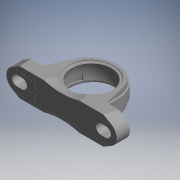
# Autodesk Inventor part: housingSYWK 506 Y-h
Saved by Autodesk Inventor 2017.3 (Build 213256000, 256)
## iProperties
Part Number: housingSYWK 506 Y-h
Material: Generic
Catalog Web Link: www.cadenas.de
Description: ayp_001_hc_hh_hy-ayl_001_hp_housing-Plummer block housings for Y-bearings
Vendor: SKF
Document SubType Name: Modeling
Designer: partserver
Manufacturer: SKF
Mass: 127.227 g
Surface Area: 312.414 cm^2
Volume: 127.227 cm^3
Density: 1 g/cm^3
Appearance: PSOLRGB-175-175-175
Category: PARTsolutions
Company: SKF
Title: housingSYWK 506 Y-h
Author: Cadenas PARTsolutions
Comments: Plummer block housings for Y-bearings
PSOL_IDENT_0: {$CADENAS_DATA\23d-libs\skf\bearings_units_and_housings\bearing_units\ball_bearing_units\y-units\y-b
PSOL_IDENT_1: earing_plummer_block_units_parts\ayp_001_hc_hh_hy-ayl_001_hp_housing.prj},217 {VTYP=3D},{NB=housingS
PSOL_IDENT_2: YWK 506 Y-h},{LINA=housingSYWK 506 Y-h},{NN=ayp_001_hc_hh_hy-ayl_001_hp_housing},{DATE=20.09.2021 12
PSOL_IDENT_3: :02:20},{GEOMDATE=16.12.2020 09:20:11},{VERSION=},{LINEID=5570},{WBVAR=ENDCOVER},{WBNUMERIC=}  {NB=h
PSOL_IDENT_4: ousingSYWK 506 Y-h},{LINA=housingSYWK 506 Y-h},{KT=DUMMY},{DESIGNATION=SYWK 506 Y},{DESIGN=sywk},{EN
PSOL_IDENT_5: DCOVER=},{ECPN=},{D=62.000},{H1=42.900},{A=40.000},{A1=25.000},{A5=30.500},{H=82.000},{H2=19.000},{J=
PSOL_IDENT_6: 121.000},{L=159.000},{N=21.500},{N1=14.500},{RG=},{R1=MIN},{RA=MIN},{DN=MIN},{SWN=MIN},{GN=},{J6=MIN
PSOL_IDENT_7: },{J7=MIN},{N4=MIN},{MASS=0.210},{G=12.000},{GIN=0.500},{COVER=ECW 206},{PIM=SYWK 506 Y},{LOOKUP=AEC
PSOL_IDENT_8: ALG,DECALG,D1ECALG,D2ECALG},{AEC=33.500},{AECALG=COVER,HEL02,AEC},{DEC=54.100},{DECALG=COVER,HED10,D
PSOL_IDENT_9: EC},{D1EC=64.400},{D1ECALG=COVER,HED13,D1EC},{D2EC=66.000},{D2ECALG=COVER,HED12,D2EC},{PPATH=apb_001
PSOL_IDENT_10: -002_apf_001_app_001_asmtpl.prj},{HIDE=0},{COPYTABLE=apb_001-002_apf_001_app_001_dummy|DUMMY,apb_001
PSOL_IDENT_11: -002_apf_001_app_001_housing|HOUSING,apb_001-002_apf_001_app_001_housing_arc|HOUSING2},{DUMMY=dummy}
PSOL_IDENT_12: ,{HOUSING=housing},{HOUSING2=housing2},{CANGLE=79.258},{ACRL=31.985},{ARCC=5.393},{S=0},{NON=},{DS=0
PSOL_IDENT_13: .000},{NOCUT=},{H3=MIN},{JMAX=128.000},{JMIN=114.000},{A5UP=31.000},{L1=MIN},{H4=MIN},{R2=MIN},{L2=M
PSOL_IDENT_14: IN},{H5=MIN},{L6=MIN},{L7=MIN},{H6=MIN},{L8=MIN},{R3=MIN},{L9=MIN},{ANG=MIN},{L10=MIN},{H7=MIN},{H8=
PSOL_IDENT_15: MIN},{R4=MIN},{R5=MIN},{R6=MIN},{H9=MIN},{ANG1=MIN},{ANG2=MIN},{L11=MIN},{R7=MIN},{L12=MIN},{R8=MIN}
PSOL_IDENT_16: ,{L13=MIN},{H10=MIN},{H11=MIN},{L14=MIN},{R9=MIN},{L15=MIN},{H12=MIN},{L16=MIN},{L17=MIN},{DRAFT=MIN
PSOL_IDENT_17: },{SCALE=MIN}
NB: housingSYWK 506 Y-h
NN: ayp_001_hc_hh_hy-ayl_001_hp_housing
NT: Plummer block housings for Y-bearings
NBSYN: $HOUSING.$DESIGNATION.$ECPN.-h
LINA: housingSYWK 506 Y-h
CATALOG: SKF
DESIGNATION: SYWK 506 Y
DESIGN: sywk
ENDCOVER: w/o End Cover
D: 62
H1: 42.9
A: 40
A1: 25
A5: 30.5
H: 82
H2: 19
J: 121
L: 159
N: 21.5
N1: 14.5
R1: 0
RA: 0
DN: 0
SWN: 0
J6: 0
J7: 0
N4: 0
MASS: 0.21
G: 12
GIN: 0.5
COVER: ECW 206
PIM: SYWK 506 Y
AEC: 33.5
DEC: 54.1
D1EC: 64.4
D2EC: 66
DS: 0
H3: 0
JMAX: 128
JMIN: 114
A5UP: 31
L1: 0
H4: 0
R2: 0
L2: 0
H5: 0
L6: 0
L7: 0
H6: 0
L8: 0
R3: 0
L9: 0
ANG: 0
L10: 0
H7: 0
H8: 0
R4: 0
R5: 0
R6: 0
H9: 0
ANG1: 0
ANG2: 0
L11: 0
R7: 0
L12: 0
R8: 0
L13: 0
H10: 0
H11: 0
L14: 0
R9: 0
L15: 0
H12: 0
L16: 0
L17: 0
DRAFT: 0
SCALE: 0
SUPPLIER: SKF
ARTICLENO: housingSYWK 506 Y-h
BOMINFO: housingSYWK 506 Y-h
CREATOR: CADENAS GmbH
Autodesk Inventor part; units mm, degrees
ref_plane "YZ Plane" through (0, 0, 0) normal (1, 0, 0) x (0, 1, 0)
ref_plane "XZ Plane" through (0, 0, 0) normal (0, 1, 0) x (-1, 0, 0)
ref_plane "XY Plane" through (0, 0, 0) normal (0, 0, 1) x (1, 0, 0)
sketch "Sketch_1" plane through (0, 0, 0) normal (1, 0, 0) x (0, 1, 0)
  line L0 (0, -20) -> (0, 20)
  line L1 (35.7991, 20) -> (32.5, 14.2857)
  line L2 (32.5, 14.2857) -> (32.5, 13.2857)
  arc A0 (31.5, 12.2857) -> (32.5, 13.2857) centre (31.5, 13.2857) ccw
  line L3 (31.5, 12.2857) -> (28.9616, 12.2857)
  line L4 (28.9616, 12.2857) -> (28.6105, 11.9347)
  arc A1 (28.6105, -11.9347) -> (28.6105, 11.9347) centre (0, 0) ccw
  line L5 (28.6105, -11.9347) -> (28.9616, -12.2857)
  line L6 (28.9616, -12.2857) -> (31.5, -12.2857)
  arc A2 (32.5, -13.2857) -> (31.5, -12.2857) centre (31.5, -13.2857) ccw
  line L7 (32.5, -13.2857) -> (32.5, -14.2857)
  line L8 (32.5, -14.2857) -> (35.7991, -20)
  line L9 (35.7991, -20) -> (119.25, -20)
  line L10 (119.25, -20) -> (119.25, 20)
  line L11 (119.25, 20) -> (35.7991, 20)
  constraints: 24 end point, 6 point on circle, 3 centre point
revolve "Revolution1" add sketch "Sketch_1" angle 360 about axis through (0, 0, -20) along (0, 0, -1)
sketch "Sketch_2" plane through (0, 0, 0) normal (0, 0, 1) x (1, 0, 0)
  circle A0 centre (0, 0) radius 119.25
  line L0 (-79.5, -23.9) -> (-79.5, -42.9)
  line L1 (-79.5, -42.9) -> (79.5, -42.9)
  line L2 (79.5, -42.9) -> (79.5, -23.9)
  line L3 (79.5, -23.9) -> (49.75, -23.9)
  arc A1 (44.9663, -20.3546) -> (49.75, -23.9) centre (49.75, -18.9) ccw
  line L4 (44.9663, -20.3546) -> (35.4954, 10.7929)
  arc A2 (35.4954, 10.7929) -> (-35.4954, 10.7929) centre (0, 0) ccw
  line L5 (-35.4954, 10.7929) -> (-44.9663, -20.3546)
  arc A3 (-49.75, -23.9) -> (-44.9663, -20.3546) centre (-49.75, -18.9) ccw
  line L6 (-49.75, -23.9) -> (-79.5, -23.9)
  constraints: 14 end point, 6 point on circle, 4 centre point
extrude "Extrusion1" cut sketch "Sketch_2" along normal mid plane 40
sketch "Sketch_3" plane through (0, 0, 0) normal (0, 1, 0) x (-1, 0, 0)
  line L0 (87.45, -22) -> (87.45, 22)
  line L1 (87.45, 22) -> (-87.45, 22)
  line L2 (-87.45, 22) -> (-87.45, -22)
  line L3 (-87.45, -22) -> (87.45, -22)
  arc A0 (71.75, -13.4234) -> (71.75, 13.4234) centre (64, 0) ccw
  line L4 (71.75, 13.4234) -> (61.5192, 19.3301)
  arc A1 (61.5192, 19.3301) -> (59.0192, 20) centre (59.0192, 15) ccw
  line L5 (59.0192, 20) -> (-59.0192, 20)
  arc A2 (-59.0192, 20) -> (-61.5192, 19.3301) centre (-59.0192, 15) ccw
  line L6 (-61.5192, 19.3301) -> (-71.75, 13.4234)
  arc A3 (-71.75, 13.4234) -> (-71.75, -13.4234) centre (-64, 0) ccw
  line L7 (-71.75, -13.4234) -> (-61.5192, -19.3301)
  arc A4 (-61.5192, -19.3301) -> (-59.0192, -20) centre (-59.0192, -15) ccw
  line L8 (-59.0192, -20) -> (59.0192, -20)
  arc A5 (59.0192, -20) -> (61.5192, -19.3301) centre (59.0192, -15) ccw
  line L9 (61.5192, -19.3301) -> (71.75, -13.4234)
  constraints: 20 end point, 12 point on circle, 6 centre point
extrude "Extrusion2" cut sketch "Sketch_3" against normal blind 42.9
sketch "Sketch_4" plane through (0, 0, 0) normal (1, 0, 0) x (0, 1, 0)
  line L0 (49.2, 24) -> (-49.2, 24)
  line L1 (-49.2, 24) -> (-49.2, -24)
  line L2 (-49.2, -24) -> (49.2, -24)
  line L3 (49.2, -24) -> (49.2, 24)
  line L4 (-42.9, 20) -> (-42.9, -20)
  line L5 (-42.9, -20) -> (39.1, -12.5)
  line L6 (39.1, -12.5) -> (39.1, 12.5)
  line L7 (39.1, 12.5) -> (-42.9, 20)
  constraints: 16 end point
extrude "Extrusion3" cut sketch "Sketch_4" along normal mid plane 159
sketch "Sketch_5" plane through (0, 0, 0) normal (1, 0, 0) x (0, 1, 0)
  line L0 (50, -109.125) -> (-50, -109.125)
  arc A0 (58.605, -109.125) -> (-127.645, -109.125) centre (-34.52, -109.125) ccw
  line L1 (58.605, -109.125) -> (-127.645, -109.125)
  constraints: 4 end point, 2 point on circle, 1 centre point
revolve "Revolution2" cut sketch "Sketch_5" angle 360 about axis through (0, 50, -109.125) along (0, 1, 0)
sketch "Sketch_6" plane through (0, 0, 0) normal (1, 0, 0) x (0, 1, 0)
  line L0 (50, 109.125) -> (-50, 109.125)
  arc A0 (58.605, 109.125) -> (-127.645, 109.125) centre (-34.52, 109.125) ccw
  line L1 (58.605, 109.125) -> (-127.645, 109.125)
  constraints: 4 end point, 2 point on circle, 1 centre point
revolve "Revolution3" cut sketch "Sketch_6" angle 360 about axis through (0, 50, 109.125) along (0, 1, 0)
sketch "Sketch_8" plane through (0, 0, 0) normal (0, 1, 0) x (-1, 0, 0)
  arc A0 (64, -7.25) -> (64, 7.25) centre (64, 0) ccw
  line L0 (64, 7.25) -> (57, 7.25)
  arc A1 (57, 7.25) -> (57, -7.25) centre (57, 0) ccw
  line L1 (57, -7.25) -> (64, -7.25)
  constraints: 4 end point, 4 point on circle, 2 centre point
extrude "Extrusion4" cut sketch "Sketch_8" against normal blind 42.9
sketch "Sketch_10" plane through (0, 0, 0) normal (0, 1, 0) x (-1, 0, 0)
  arc A0 (-57, -7.25) -> (-57, 7.25) centre (-57, 0) ccw
  line L0 (-57, 7.25) -> (-64, 7.25)
  arc A1 (-64, 7.25) -> (-64, -7.25) centre (-64, 0) ccw
  line L1 (-64, -7.25) -> (-57, -7.25)
  constraints: 4 end point, 4 point on circle, 2 centre point
extrude "Extrusion5" cut sketch "Sketch_10" against normal blind 42.9
sketch "Sketch_11" plane through (0, 0, 0) normal (0, 1, 0) x (-1, 0, 0)
  line L0 (60.5, 15.4) -> (38.1, 15.4)
  arc A0 (38.1, 15.4) -> (37.1, 14.4) centre (38.1, 14.4) ccw
  line L1 (37.1, 14.4) -> (37.1, -14.4)
  arc A1 (37.1, -14.4) -> (38.1, -15.4) centre (38.1, -14.4) ccw
  line L2 (38.1, -15.4) -> (60.5, -15.4)
  line L3 (60.5, -15.4) -> (60.5, 15.4)
  constraints: 8 end point, 4 point on circle, 2 centre point
extrude "Extrusion6" cut sketch "Sketch_11" along normal mid plane 47.8
sketch "Sketch_7" plane through (0, 0, 0) normal (0, 1, 0) x (-1, 0, 0)
  line L0 (-37.1, -14.6) -> (-37.1, 14.6)
  arc A0 (-37.1, 14.6) -> (-38.1, 15.6) centre (-38.1, 14.6) ccw
  line L1 (-38.1, 15.6) -> (-60.5, 15.6)
  line L2 (-60.5, 15.6) -> (-60.5, -15.6)
  line L3 (-60.5, -15.6) -> (-38.1, -15.6)
  arc A1 (-38.1, -15.6) -> (-37.1, -14.6) centre (-38.1, -14.6) ccw
  constraints: 8 end point, 4 point on circle, 2 centre point
extrude "Extrusion7" cut sketch "Sketch_7" along normal mid plane 47.8
sketch "Sketch_9" plane through (0, 0, 0) normal (1, 0, 0) x (0, 1, 0)
  line L0 (0, -20) -> (0, 20)
  line L1 (38.1, 8.75) -> (37.1, 8.75)
  line L2 (37.1, 8.75) -> (37.1, -8.75)
  line L3 (37.1, -8.75) -> (38.1, -8.75)
  arc A0 (38.1, -8.75) -> (39.1, -7.75) centre (38.1, -7.75) ccw
  line L4 (39.1, -7.75) -> (39.1, 7.75)
  arc A1 (39.1, 7.75) -> (38.1, 8.75) centre (38.1, 7.75) ccw
  constraints: 10 end point, 4 point on circle, 2 centre point
revolve "Revolution4" add sketch "Sketch_9" angle 180 mid plane about axis through (0, 0, -20) along (0, 0, 1)
sketch "Sketch_12" plane through (0, 0, 0) normal (0, 1, 0) x (-1, 0, 0)
  line L0 (-37.1, -8.75) -> (-37.1, 8.75)
  line L1 (-37.1, 8.75) -> (-38.1, 8.75)
  arc A0 (-38.1, 8.75) -> (-39.1, 7.75) centre (-38.1, 7.75) ccw
  line L2 (-39.1, 7.75) -> (-39.1, -7.75)
  arc A1 (-39.1, -7.75) -> (-38.1, -8.75) centre (-38.1, -7.75) ccw
  line L3 (-38.1, -8.75) -> (-37.1, -8.75)
  constraints: 8 end point, 4 point on circle, 2 centre point
extrude "Extrusion8" add sketch "Sketch_12" against normal blind 42.9
sketch "Sketch_19" plane through (0, 0, 0) normal (0, 1, 0) x (-1, 0, 0)
  line L0 (39.1, -7.75) -> (39.1, 7.75)
  arc A0 (39.1, 7.75) -> (38.1, 8.75) centre (38.1, 7.75) ccw
  line L1 (38.1, 8.75) -> (37.1, 8.75)
  line L2 (37.1, 8.75) -> (37.1, -8.75)
  line L3 (37.1, -8.75) -> (38.1, -8.75)
  arc A1 (38.1, -8.75) -> (39.1, -7.75) centre (38.1, -7.75) ccw
  constraints: 8 end point, 4 point on circle, 2 centre point
extrude "Extrusion9" add sketch "Sketch_19" against normal blind 42.9
sketch "Sketch_13" plane through (0, 0, -1) normal (0, 0, 1) x (1, 0, 0)
  arc A0 (-27.8332, 14.75) -> (-27.8332, -14.75) centre (0, 0) ccw
  line L0 (-27.8332, -14.75) -> (27.8332, -14.75)
  arc A1 (27.8332, -14.75) -> (27.8332, 14.75) centre (0, 0) ccw
  line L1 (27.8332, 14.75) -> (-27.8332, 14.75)
  constraints: 4 end point, 4 point on circle, 2 centre point
extrude "Extrusion10" cut sketch "Sketch_13" along normal blind 21
sketch "Sketch_14" plane through (0, 0, 0) normal (0, 1, 0) x (-1, 0, 0)
  line L0 (0, 9.5) -> (0, 47)
  line L1 (0, 47) -> (22.2204, 47)
  arc A0 (27.05, 43.2941) -> (22.2204, 47) centre (22.2204, 42) ccw
  line L2 (27.05, 43.2941) -> (31.1298, 28.068)
  arc A1 (32.1338, 21.3504) -> (31.1298, 28.068) centre (2.152, 20.3034) ccw
  line L3 (32.1338, 21.3504) -> (32.4162, 13.2612)
  line L4 (32.4162, 13.2612) -> (32.2, 11.5)
  line L5 (32.2, 11.5) -> (32.7037, 11.134)
  arc A2 (32.9742, 10.7257) -> (32.7037, 11.134) centre (32.2923, 10.5677) ccw
  arc A3 (32, 9.5) -> (32.9742, 10.7257) centre (32, 10.5) ccw
  line L6 (32, 9.5) -> (0, 9.5)
  line L7 (0, 9.5) -> (0, 47)
  constraints: 16 end point, 8 point on circle, 4 centre point
revolve "Revolution5" cut sketch "Sketch_14" angle 360 about axis through (0, 0, 9.5) along (0, 0, -1)
sketch "Sketch_21" plane through (0, -42.9, 0) normal (0, 1, 0) x (1, 0, 0)
  arc A0 (-63.6368, -12.9995) -> (-64.3439, -14.7066) centre (-63.6368, -13.9995) ccw
  line L0 (-64.3439, -14.7066) -> (-63.844, -15.2065)
  line L1 (-63.844, -15.2065) -> (-63.137, -15.4995)
  line L2 (-63.137, -15.4995) -> (-36.675, -15.4995)
  arc A1 (-36.675, -15.4995) -> (-36.8933, -13.9389) centre (-37.394, -14.8045) ccw
  line L3 (-36.8933, -13.9389) -> (-37.653, -13.4995)
  line L4 (-37.653, -13.4995) -> (-36.187, -13.4995)
  line L5 (-36.187, -13.4995) -> (-36.187, -15.3945)
  line L6 (-36.187, -15.3945) -> (-35.662, -17.8385)
  arc A2 (36.587, -17.8385) -> (-35.662, -17.8385) centre (0.4625, -185.903) ccw
  line L7 (36.587, -17.8385) -> (37.113, -15.3945)
  line L8 (37.113, -15.3945) -> (37.113, -13.4995)
  line L9 (37.113, -13.4995) -> (38.578, -13.4995)
  line L10 (38.578, -13.4995) -> (37.819, -13.9385)
  arc A3 (37.819, -13.9385) -> (37.601, -15.4995) centre (38.3197, -14.8041) ccw
  line L11 (37.601, -15.4995) -> (64.063, -15.4995)
  line L12 (64.063, -15.4995) -> (64.77, -15.2065)
  line L13 (64.77, -15.2065) -> (65.2699, -14.7066)
  arc A4 (65.2699, -14.7066) -> (64.5628, -12.9995) centre (64.5628, -13.9995) ccw
  line L14 (64.5628, -12.9995) -> (57.463, -12.9995)
  arc A5 (48.02, -8.9355) -> (57.463, -12.9995) centre (57.4618, 0.0005) ccw
  line L15 (48.02, -8.9355) -> (46.794, -8.7565)
  line L16 (46.794, -8.7565) -> (43.774, -10.4995)
  line L17 (43.774, -10.4995) -> (37.113, -10.4995)
  line L18 (37.113, -10.4995) -> (37.113, -3.4995)
  line L19 (37.113, -3.4995) -> (43.688, -3.4995)
  arc A6 (43.688, -3.4995) -> (44.672, -2.3215) centre (43.688, -2.4995) ccw
  arc A7 (44.672, 2.3215) -> (44.672, -2.3215) centre (57.463, 0) ccw
  arc A8 (44.672, 2.3215) -> (43.6882, 3.5005) centre (43.6882, 2.5005) ccw
  line L20 (43.6882, 3.5005) -> (37.113, 3.5005)
  line L21 (37.113, 3.5005) -> (37.113, 10.5005)
  line L22 (37.113, 10.5005) -> (43.774, 10.5005)
  line L23 (43.774, 10.5005) -> (46.794, 8.7565)
  line L24 (46.794, 8.7565) -> (48.02, 8.9355)
  arc A9 (57.4628, 13.0005) -> (48.02, 8.9355) centre (57.4628, 0.0005) ccw
  line L25 (57.4628, 13.0005) -> (64.5628, 13.0005)
  arc A10 (64.5628, 13.0005) -> (65.2699, 14.7076) centre (64.5628, 14.0005) ccw
  line L26 (65.2699, 14.7076) -> (64.77, 15.2075)
  line L27 (64.77, 15.2075) -> (64.063, 15.5005)
  line L28 (64.063, 15.5005) -> (37.601, 15.5005)
  arc A11 (37.601, 15.5005) -> (37.8192, 13.9384) centre (38.319, 14.8045) ccw
  line L29 (37.8192, 13.9384) -> (38.578, 13.5005)
  line L30 (38.578, 13.5005) -> (37.113, 13.5005)
  line L31 (37.113, 13.5005) -> (37.113, 15.3945)
  line L32 (37.113, 15.3945) -> (36.587, 17.8385)
  arc A12 (-35.662, 17.8385) -> (36.587, 17.8385) centre (0.4625, 185.903) ccw
  line L33 (-35.662, 17.8385) -> (-36.187, 15.3945)
  line L34 (-36.187, 15.3945) -> (-36.187, 13.5005)
  line L35 (-36.187, 13.5005) -> (-37.653, 13.5005)
  line L36 (-37.653, 13.5005) -> (-36.8936, 13.9387)
  arc A13 (-36.8936, 13.9387) -> (-36.675, 15.5005) centre (-37.3934, 14.8049) ccw
  line L37 (-36.675, 15.5005) -> (-63.137, 15.5005)
  line L38 (-63.137, 15.5005) -> (-63.844, 15.2075)
  line L39 (-63.844, 15.2075) -> (-64.3439, 14.7076)
  arc A14 (-64.3439, 14.7076) -> (-63.6368, 13.0005) centre (-63.6368, 14.0005) ccw
  line L40 (-63.6368, 13.0005) -> (-56.5378, 13.0005)
  arc A15 (-47.095, 8.9355) -> (-56.5378, 13.0005) centre (-56.5378, 0.0005) ccw
  line L41 (-47.095, 8.9355) -> (-45.869, 8.7565)
  line L42 (-45.869, 8.7565) -> (-42.849, 10.5005)
  line L43 (-42.849, 10.5005) -> (-36.187, 10.5005)
  line L44 (-36.187, 10.5005) -> (-36.187, 3.5005)
  line L45 (-36.187, 3.5005) -> (-42.7622, 3.5005)
  arc A16 (-42.7622, 3.5005) -> (-43.746, 2.3215) centre (-42.7622, 2.5005) ccw
  arc A17 (-43.746, -2.3215) -> (-43.746, 2.3215) centre (-56.537, 0) ccw
  arc A18 (-43.746, -2.3215) -> (-42.762, -3.4995) centre (-42.762, -2.4995) ccw
  line L46 (-42.762, -3.4995) -> (-36.187, -3.4995)
  line L47 (-36.187, -3.4995) -> (-36.187, -10.4995)
  line L48 (-36.187, -10.4995) -> (-42.849, -10.4995)
  line L49 (-42.849, -10.4995) -> (-45.869, -8.7565)
  line L50 (-45.869, -8.7565) -> (-47.095, -8.9355)
  arc A19 (-56.5368, -12.9995) -> (-47.095, -8.9355) centre (-56.5368, 0.0005) ccw
  line L51 (-56.5368, -12.9995) -> (-63.6368, -12.9995)
  constraints: 104 end point, 40 point on circle, 20 centre point
extrude "Extrusion11" cut sketch "Sketch_21" along normal blind 0.1
ref_plane "brg_XY" through (0, 0, 0) normal (0, 0, 1) x (1, 0, 0)
ref_plane "brg_YZ" through (0, 0, 0) normal (1, 0, 0) x (0, 1, 0)
ref_plane "brg_ZX" through (0, 0, 0) normal (0, 1, 0) x (0, 0, 1)
ref_plane "housing_XY" through (0, -42.9, 0) normal (0, 1, 0) x (1, 0, 0)
ref_plane "housing_YZ" through (0, -42.9, 0) normal (1, 0, 0) x (0, 0, -1)
ref_plane "housing_ZX" through (0, -42.9, 0) normal (0, 0, -1) x (0, 1, 0)
ref_plane "tocover_XY" through (0, 0, 43) normal (0, 0, 1) x (1, 0, 0)
ref_plane "tocover_YZ" through (0, 0, 43) normal (1, 0, 0) x (0, 1, 0)
ref_plane "tocover_ZX" through (0, 0, 43) normal (0, 1, 0) x (0, 0, 1)
body "Solid1"
